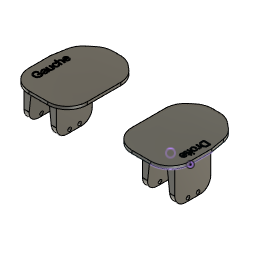
Sensor case - support (Autodesk Fusion 360 design; units mm, degrees)
Autodesk Fusion 360 part; units mm, degrees
sketch "Sketch3" plane through (0, 0, 0) normal (0, 0, 1) x (1, 0, 0)
  circle A0 centre (0, 0) radius 500 construction
  line L0 (-15, 41.2122) -> (-37.9813, 21.9285)
  line L1 (37.9813, 21.9285) -> (43.1908, -7.6157)
  line L2 (0, 0) -> (-321.3938, 383.0222) construction
  line L3 (0, 0) -> (492.4039, 86.8241) construction
  line L4 (37.9813, 21.9285) -> (15, 41.2122)
  line L5 (15, 41.2122) -> (-15, 41.2122)
  line L6 (0, 0) -> (321.3938, 383.0222) construction
  line L7 (0, 0) -> (-470, 0) construction
  line L8 (0, 0) -> (0, 500) construction
  line L9 (-37.9813, 21.9285) -> (-37.9813, -65.0715)
  line L10 (0, 0) -> (0, -60.871) construction
  line L11 (-37.9813, -65.0715) -> (12.0187, -65.0715)
  line L12 (12.0187, -65.0715) -> (43.1908, -65.0715)
  line L13 (43.1908, -65.0715) -> (43.1908, -7.6157)
  dimension "d12" = 470
  dimension "d13" = 40
  dimension "d14" = 40
  dimension "d15" = 40
  dimension "d16" = 1000
  dimension "d17" = 30
  dimension "d18" = 15
  dimension "d19" = 15
  dimension "d21" = 10
  dimension "d111" = 87
  constraint coincident A0.centre L2.start
  constraint horizontal L7
  constraint coincident L8.end A0
  constraint coincident L2.end A0
  constraint coincident L3.end A0
  constraint coincident L6.end A0
  constraint equal L4 L5
  constraint equal L0 L5
  constraint perpendicular L5 L8
  constraint perpendicular L0 L2
  constraint perpendicular L4 L6
  constraint equal L1 L4
  constraint perpendicular L1 L3
  constraint perpendicular L10 L11
  constraint perpendicular L7 L9
  constraint perpendicular L9 L11
  constraint parallel L11 L12
  constraint perpendicular L12 L13
  measures "d12" distance of A0.centre L7.end
  measures "d13" angle of L3 L6
  measures "d14" angle of L6 L8
  measures "d15" angle of L2 L8
  measures "d16" diameter of A0
  measures "d17" distance of L1.start L4.end
  measures "d18" distance of L1.start L6
  measures "d19" distance of L0.start L2
  measures "d21" angle of L3 L7
  measures "d111" distance of L0.end L9.end
extrude "Extrude16" add sketch "Sketch3" along normal blind 2 makes body 1
sketch "Sketch19" plane through (0, 0, 0) normal (0, 0, -1) x (1, 0, 0)
  line L0 (15, -41.2122) -> (37.9813, -21.9285)
  line L1 (37.9813, -21.9285) -> (43.1908, 7.6157)
  line L2 (43.1908, 65.0715) -> (-37.9813, 65.0715)
  line L3 (-37.9813, 65.0715) -> (-37.9813, -21.9285)
  line L4 (-37.9813, -21.9285) -> (-15, -41.2122)
  line L5 (-15, -41.2122) -> (15, -41.2122)
  line L6 (40.1908, 11.7878) -> (43.1908, 11.7878)
  line L7 (43.1908, 11.7878) -> (43.1908, 65.0715)
  line L8 (43.1908, 65.0715) -> (40.1908, 65.0715)
  line L9 (40.1908, 65.0715) -> (40.1908, 11.7878)
  line L10 (43.1908, 7.6157) -> (43.1908, 65.0715)
  dimension "d119" = 3
  dimension "d143" = 53
  constraint horizontal L6
  constraint vertical L7
  constraint horizontal L8
  constraint vertical L9
  constraint collinear L2 L8
  constraint coincident L2.start L7.end
  measures "d119" distance of L7 L9
  measures "d143" distance of L5 L6
fillet "Fillet10" radius 27.5 6 edges at (-15, 41.2122, 1) (15, 41.2122, 1) (37.9813, 21.9285, 1) (-37.9813, 21.9285, 1) (-37.9813, -65.0715, 1) (43.1908, -65.0715, 1) on bodies 1
sketch "Esquisse31" plane through (0, 0, 0) normal (0, 0, -1) x (1, 0, 0)
  arc A0 (-10.4813, 65.0715) -> (-37.9813, 37.5715) centre (-10.4813, 37.5715) ccw
  line L0 (-37.9813, 37.5715) -> (-37.9813, -9.1051)
  arc A1 (-37.9813, -9.1051) -> (-28.158, -30.1713) centre (-10.4813, -9.1051) ccw
  line L1 (-28.158, -30.1713) -> (-22.6675, -34.7784)
  arc A2 (-22.6675, -34.7784) -> (-4.9908, -41.2122) centre (-4.9908, -13.7122) ccw
  line L2 (-4.9908, -41.2122) -> (4.9908, -41.2122)
  arc A3 (4.9908, -41.2122) -> (22.6675, -34.7784) centre (4.9908, -13.7122) ccw
  line L3 (22.6675, -34.7784) -> (30.3139, -28.3623)
  arc A4 (30.3139, -28.3623) -> (39.7194, -12.0714) centre (12.6372, -7.2961) ccw
  line L4 (39.7194, -12.0714) -> (43.1908, 7.6157)
  line L5 (15.6908, 65.0715) -> (-10.4813, 65.0715)
  line L6 (43.1908, 7.6157) -> (43.1908, 37.5715)
  arc A5 (43.1908, 37.5715) -> (15.6908, 65.0715) centre (15.6908, 37.5715) ccw
sketch "Esquisse32" plane through (0, 0, 0) normal (0, 0, -1) x (1, 0, 0)
  line L0 (-9.1283, 51.7334) -> (35.8717, 51.7334)
  line L1 (35.8717, 51.7334) -> (35.8717, 1.7334)
  line L2 (35.8717, 1.7334) -> (-9.1283, 1.7334)
  line L3 (-9.1283, 1.7334) -> (-9.1283, 51.7334)
  dimension "d190" = 50
  dimension "d191" = 45
  constraint horizontal L0
  constraint vertical L1
  constraint horizontal L2
  constraint vertical L3
  measures "d190" distance of L0 L2
  measures "d191" distance of L0.start L0.end
extrude "Extrusion30" add sketch "Esquisse32" along normal blind 50 bodies 1
sketch "Esquisse33" plane through (0, -51.7334, 0) normal (0, -1, 0) x (1, 0, 0)
  line L0 (35.8717, 0) -> (-9.1283, 0)
  line L1 (-9.1283, 0) -> (-9.1283, -50)
  line L2 (-9.1283, -50) -> (35.8717, -50)
  line L3 (35.8717, -50) -> (35.8717, 0)
  line L4 (-3.6283, -50) -> (0.8717, -10)
  arc A0 (25.8717, -10) -> (0.8717, -10) centre (13.3717, -11.4063) ccw
  line L5 (25.8717, -10) -> (30.3717, -50)
  line L6 (-21.5939, -10) -> (55.3736, -10) construction
  line L7 (15.6908, 0) -> (43.1908, 0) construction
  line L8 (13.3717, -4.8712) -> (13.3717, -95.1288) construction
  dimension "d194" = 34
  dimension "d195" = 25
  dimension "d196" = 10
  dimension "d197" = 17
  constraint coincident L2 L4.start
  constraint tangent L4 A0
  constraint coincident L2 L5.end
  constraint tangent A0 L5
  constraint perpendicular L1 L6
  constraint coincident A0.start L6
  constraint coincident L4.end L6
  constraint vertical L8
  constraint midpoint L2 L8
  measures "d194" distance of L4.start L5.end
  measures "d195" distance of L4.end A0.start
  measures "d196" distance of L6 L7
  measures "d197" distance of L4.start L8
extrude "Extrusion31" cut sketch "Esquisse33" against normal up to surface (50 mm away) contours L0 L2 L4 A0 L5 bodies 1
fillet "Congé11" radius 15 4 edges at (33.1217, -51.7334, -50) (33.1217, -1.7334, -50) (-6.3783, -1.7334, -50) (-6.3783, -51.7334, -50) on bodies 1
sketch "Esquisse34" plane through (-9.1283, 0, 0) normal (-1, 0, 0) x (0, -1, 0)
  arc A0 (36.7334, -50) -> (51.7334, -35) centre (36.7334, -35) ccw
  line L0 (51.7334, -35) -> (51.7334, 0)
  line L1 (51.7334, 0) -> (1.7334, 0)
  line L2 (1.7334, 0) -> (1.7334, -35)
  arc A1 (1.7334, -35) -> (16.7334, -50) centre (16.7334, -35) ccw
  line L3 (16.7334, -50) -> (36.7334, -50)
  circle A2 centre (19.2166, -46) radius 2.5
  circle A3 centre (33.2582, -46) radius 2.5
  point P0 (36.7334, -50)
  dimension "d202" = 5
  dimension "d203" = 4
  dimension "d204" = 5
  dimension "d205" = 4
  measures "d202" diameter of A2
  measures "d203" distance of L3 A2.centre
  measures "d204" diameter of A3
  measures "d205" distance of L3 A3.centre
extrude "Extrusion32" cut sketch "Esquisse34" against normal up to surface (45 mm away) contours A2 | A3 bodies 1
extrude "Extrusion33" add 1 faces at (-10.924, -12.0274, 2) along direction (0, 0, 1) blind 2 on bodies 1 bodies 1
ref_plane "Plan de construction1" through (-69.1283, -26.7334, -25) normal (-1, 0, 0) x (0, 1, 0)
mirror "Symétrie miroir1" about plane through (-69.1283, -26.7334, -25) normal (-1, 0, 0) of bodies 1 makes body 2
sketch "Esquisse36" plane through (0, 0, 4) normal (0, 0, 1) x (-1, 0, 0)
  arc A0 (-15.6908, 65.0715) -> (-43.1908, 37.5715) centre (-15.6908, 37.5715) ccw
  line L0 (-43.1908, 37.5715) -> (-43.1908, 7.6157)
  line L1 (-43.1908, 7.6157) -> (-39.7194, -12.0714)
  arc A1 (-39.7194, -12.0714) -> (-30.3139, -28.3623) centre (-12.6372, -7.2961) ccw
  line L2 (-30.3139, -28.3623) -> (-22.6675, -34.7784)
  arc A2 (-22.6675, -34.7784) -> (-4.9908, -41.2122) centre (-4.9908, -13.7122) ccw
  line L3 (-4.9908, -41.2122) -> (4.9908, -41.2122)
  arc A3 (4.9908, -41.2122) -> (22.6675, -34.7784) centre (4.9908, -13.7122) ccw
  line L4 (22.6675, -34.7784) -> (28.158, -30.1713)
  arc A4 (28.158, -30.1713) -> (37.9813, -9.1051) centre (10.4813, -9.1051) ccw
  line L5 (37.9813, -9.1051) -> (37.9813, 37.5715)
  arc A5 (37.9813, 37.5715) -> (10.4813, 65.0715) centre (10.4813, 37.5715) ccw
  line L6 (10.4813, 65.0715) -> (-15.6908, 65.0715)
  line L7 (2.8507, -16.7075) -> (2.8507, 38.4421) construction
  line L8 (2.8507, 38.4421) -> (-37.2581, 38.4421) construction
  line L9 (-37.2581, 38.4421) -> (-37.2581, -16.7075) construction
  line L10 (-37.2581, -16.7075) -> (2.8507, -16.7075) construction
  dimension "d213" = 10
  text T0 "Droite" font "Arial" height 10 align right top in box 55.1496 x 40.1088 at (2.8507, -16.7075) x (0, 1) y (-1, 0) spacing 1 kerned
sketch "Esquisse37" plane through (0, 0, 4) normal (0, 0, 1) x (-1, 0, 0)
  arc A0 (181.4474, 37.5715) -> (153.9474, 65.0715) centre (153.9474, 37.5715) ccw
  line L0 (153.9474, 65.0715) -> (127.7753, 65.0715)
  arc A1 (127.7753, 65.0715) -> (100.2753, 37.5715) centre (127.7753, 37.5715) ccw
  line L1 (100.2753, 37.5715) -> (100.2753, -9.1051)
  arc A2 (100.2753, -9.1051) -> (110.0986, -30.1713) centre (127.7753, -9.1051) ccw
  line L2 (110.0986, -30.1713) -> (115.5891, -34.7784)
  arc A3 (115.5891, -34.7784) -> (133.2658, -41.2122) centre (133.2658, -13.7122) ccw
  line L3 (133.2658, -41.2122) -> (143.2474, -41.2122)
  arc A4 (143.2474, -41.2122) -> (160.9241, -34.7784) centre (143.2474, -13.7122) ccw
  line L4 (160.9241, -34.7784) -> (168.5704, -28.3623)
  arc A5 (168.5704, -28.3623) -> (177.976, -12.0714) centre (150.8938, -7.2961) ccw
  line L5 (177.976, -12.0714) -> (181.4474, 7.6157)
  line L6 (181.4474, 7.6157) -> (181.4474, 37.5715)
  line L7 (144.2601, 61.7008) -> (144.2601, -3.2254) construction
  line L8 (144.2601, -3.2254) -> (173.0987, -3.2254) construction
  line L9 (173.0987, -3.2254) -> (173.0987, 61.7008) construction
  line L10 (173.0987, 61.7008) -> (144.2601, 61.7008) construction
  dimension "d214" = 10
  text T0 "Gauche" font "Arial" height 10 align right top in box 64.9262 x 28.8386 at (144.2601, 61.7008) x (0, -1) y (1, 0) spacing 1
emboss "Gravure en relief1" depth -0.5 profiles "Esquisse37" section 1 text T0 onto face at (-127.3326, -12.0274, 4) on bodies 2 bodies 2
emboss "Gravure en relief2" depth -0.5 profiles "Esquisse36" section 1 text T0 onto face at (-10.924, -12.0274, 4) on bodies 1 bodies 1
equation "d197 = d194 / 2"
